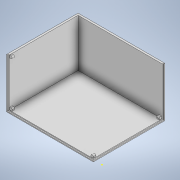
# Autodesk Inventor part: kevnat part1
Saved by Autodesk Inventor 2022 (Build 260153000, 153)
## iProperties
Created: 2023-03-07
Part Number: kevnat part1
Material: Generic
Document SubType Name: Modeling
Designer: Riordan
Density: 1 g/cm^3
Appearance: Default
Author: Riordan
Autodesk Inventor part; units mm, degrees
ref_plane "YZ Plane" through (0, 0, 0) normal (1, 0, 0) x (0, 1, 0)
ref_plane "XZ Plane" through (0, 0, 0) normal (0, 1, 0) x (-1, 0, 0)
sketch "Sketch1" plane through (0, 0, 0) normal (0, 1, 0) x (-1, 0, 0)
  line L0 (0, 0) -> (200, 0)
  line L1 (200, 0) -> (200, -150)
  line L2 (200, -150) -> (0, -150)
  line L3 (0, -150) -> (0, 0)
  dimension "d0" = 200
  dimension "d1" = 150
  constraints: 8 end point, 2 parallel, 1 horizontal, 1 perpendicular
  measures "d0" distance of L1.end L2.end
  measures "d1" distance of L0.end L1.end
extrude "Extrusion1" add sketch "Sketch1" along normal blind 2
sketch "Sketch2" plane through (0, 2, 0) normal (0, 1, 0) x (1, 0, 0)
  line L0 (-200, 0) -> (0, 0) projected
  line L1 (-200, 0) -> (-200, 2)
  line L2 (-200, 150) -> (-200, 0) projected
  line L3 (-200, 2) -> (-2, 2)
  line L4 (-2, 2) -> (-2, 150)
  line L5 (0, 150) -> (-200, 150) projected
  line L6 (-200, 2) -> (-200, 150)
  line L7 (-200, 150) -> (-2, 150)
  dimension "d4" = 2
  dimension "d5" = 198
  constraints: 10 end point, 3 perpendicular, 3 point on line
  measures "d4" distance of L0.start L1.end
  measures "d5" distance of L1.end L3.end
extrude "Extrusion2" add sketch "Sketch2" along normal blind 2
sketch "Sketch3" plane through (0, 4, 0) normal (0, 1, 0) x (1, 0, 0)
  line L0 (0, 0) -> (0, 150) projected
  line L1 (0, 0) -> (-198, 0)
  line L2 (-198, 0) -> (-198, 148)
  line L3 (-198, 148) -> (0, 148)
  line L4 (0, 148) -> (0, 0)
  line L5 (0, 150) -> (-200, 150) projected
  line L6 (-200, 150) -> (0, 150)
  line L7 (0, 150) -> (0, 0)
  line L8 (0, 0) -> (-200, 0)
  line L9 (-200, 0) -> (-200, 150)
  dimension "d8" = 198
  dimension "d9" = 148
  constraints: 16 end point, 4 parallel, 2 horizontal, 2 perpendicular
  measures "d8" distance of L2.end L3.end
  measures "d9" distance of L1.end L2.end
extrude "Extrusion3" add sketch "Sketch3" along normal blind 100 and the other way blind 2 contours L3 L2 L8 L9 L5 L0
sketch "Sketch4" plane through (0, 4, 0) normal (0, 1, 0) x (1, 0, 0)
  line L0 (-198, 2) -> (-2, 2) projected
  line L1 (-198, 2) -> (-196, 2)
  line L2 (-196, 2) -> (-196, 146)
  line L3 (-2, 148) -> (-198, 148) projected
  line L4 (-196, 146) -> (-2, 146)
  line L5 (-2, 2) -> (-2, 148) projected
  line L6 (-2, 2) -> (-198, 2)
  line L7 (-198, 2) -> (-198, 148)
  line L8 (-198, 148) -> (-2, 148)
  line L9 (-2, 148) -> (-2, 2)
  point P0 (0, 0)
  dimension "d14" = 2
  dimension "d15" = 144
  constraints: 14 end point, 3 perpendicular, 2 parallel, 2 point on line, 1 horizontal
  measures "d14" distance of L0.start L1.end
  measures "d15" distance of L1.end L2.end
extrude "Extrusion4" add sketch "Sketch4" along normal blind 100 contours L7 L3 L5 L4 L2 L0
sketch "Sketch7" plane through (0, 4, 0) normal (0, 1, 0) x (1, 0, 0)
  line L0 (-196, 2) -> (-2, 2) projected
  line L1 (-196, 2) -> (-196, 3)
  line L2 (-196, 146) -> (-196, 2) projected
  line L3 (-196, 3) -> (-191, 3)
  line L4 (-191, 3) -> (-191, 8)
  line L5 (-191, 8) -> (-196, 8)
  point P0 (0, 0)
  point P1 (-196, 117.9293)
  dimension "d36" = 1
  dimension "d37" = 5
  dimension "d38" = 5
  constraints: 8 end point, 3 perpendicular, 2 point on line
  measures "d36" distance of L0.start L1.end
  measures "d37" distance of L1.end L3.end
  measures "d38" distance of L3.end L4.end
extrude "Extrusion7" add sketch "Sketch7" along normal blind 5
fillet "Fillet2" radius 2.5 1 edges at (-191, 9, -5.5)
sketch "Sketch9" plane through (0, 4, 0) normal (0, 1, 0) x (1, 0, 0)
  line L0 (-196, 2) -> (-2, 2) projected
  line L1 (-2, 2) -> (-2, 3)
  line L2 (-2, 2) -> (-2, 146) projected
  line L3 (-2, 3) -> (-3, 3)
  line L4 (-3, 3) -> (-8, 3)
  line L5 (-8, 3) -> (-8, 8)
  line L6 (-8, 8) -> (-3, 8)
  line L7 (-3, 8) -> (-3, 3)
  point P0 (0, 0)
  dimension "d45" = 1
  dimension "d46" = 1
  dimension "d47" = 5
  dimension "d48" = 5
  constraints: 12 end point, 2 horizontal, 2 parallel, 1 perpendicular, 1 point on line
  measures "d45" distance of L0.end L1.end
  measures "d46" distance of L1.end L3.end
  measures "d47" distance of L5.end L6.end
  measures "d48" distance of L4.end L5.end
extrude "Extrusion9" add sketch "Sketch9" along normal blind 5
fillet "Fillet3" radius 2.5 2 edges at (-8, 9, -5.5) (-3, 9, -5.5)
sketch "Sketch10" plane through (-8, 4, -3) normal (0, 0, 1) x (1, 0, 0)
  arc A0 (5, 2.5) -> (0, 2.5) centre (2.5, 2.5) ccw projected
  circle A1 centre (2.5, 2.5) radius 1
  point P0 (8, -4)
  dimension "d52" = 2
  constraints: 1 centre point, 1 coincident
  measures "d52" diameter of A1
extrude "Extrusion10" cut sketch "Sketch10" against normal blind 5
sketch "Sketch11" plane through (0, 4, 0) normal (0, 1, 0) x (1, 0, 0)
  line L0 (-2, 146) -> (-196, 146) projected
  line L1 (-2, 146) -> (-3, 146)
  line L2 (-3, 146) -> (-8, 146)
  line L3 (-8, 146) -> (-8, 141)
  line L4 (-8, 141) -> (-3, 141)
  line L5 (-3, 141) -> (-3, 146)
  point P0 (0, 0)
  point P1 (-144.9293, 146)
  dimension "d55" = 1
  dimension "d56" = 5
  dimension "d57" = 5
  constraints: 10 end point, 2 parallel, 1 horizontal, 1 perpendicular, 1 point on line
  measures "d55" distance of L0.start L1.end
  measures "d56" distance of L4.end L3.end
  measures "d57" distance of L3.end L2.end
extrude "Extrusion11" add sketch "Sketch11" along normal blind 5
fillet "Fillet4" radius 2.5 1 edges at (-5.5, 9, -141)
sketch "Sketch12" plane through (-3, 4, -141) normal (1, 0, 0) x (0, 0, -1)
  arc A0 (2.5, 5) -> (0, 2.5) centre (2.5, 2.5) ccw projected
  circle A1 centre (2.5, 2.5) radius 1
  point P0 (-141, -4)
  dimension "d61" = 2
  constraints: 1 centre point, 1 coincident
  measures "d61" diameter of A1
extrude "Extrusion12" cut sketch "Sketch12" against normal blind 5
sketch "Sketch13" plane through (-196, 104, -146) normal (0, 0, 1) x (1, 0, 0)
  line L0 (0, 0) -> (194, 0) projected
  line L1 (194, 0) -> (193, 0)
  line L2 (193, 0) -> (193, -1)
  line L3 (193, -1) -> (188, -1)
  line L4 (188, -1) -> (188, -6)
  line L5 (188, -6) -> (193, -6)
  line L6 (193, -6) -> (193, -1)
  point P0 (196, -104)
  dimension "d64" = 1
  dimension "d65" = 1
  dimension "d66" = 5
  dimension "d67" = 5
  constraints: 12 end point, 2 parallel, 2 perpendicular, 1 horizontal, 1 point on line
  measures "d64" distance of L0.end L1.end
  measures "d65" distance of L1.end L2.end
  measures "d66" distance of L5.end L4.end
  measures "d67" distance of L4.end L3.end
extrude "Extrusion13" add sketch "Sketch13" along normal blind 5
fillet "Fillet5" radius 2.5 2 edges at (-5.5, 103, -141) (-5.5, 98, -141)
sketch "Sketch14" plane through (-3, 98, -146) normal (1, 0, 0) x (0, 0, -1)
  arc A0 (-2.5, 5) -> (-2.5, 0) centre (-2.5, 2.5) ccw projected
  circle A1 centre (-2.5, 2.5) radius 1
  point P0 (-146, -98)
  dimension "d71" = 2
  constraints: 1 centre point, 1 coincident
  measures "d71" diameter of A1
extrude "Extrusion14" cut sketch "Sketch14" against normal blind 5
sketch "Sketch15" plane through (-196, 4, -2) normal (1, 0, 0) x (0, 0, -1)
  line L0 (0, 100) -> (0, -2) projected
  line L1 (0, 100) -> (1, 100)
  line L2 (148, 100) -> (-2, 100) projected
  line L3 (1, 100) -> (1, 99)
  line L4 (1, 99) -> (6, 99)
  line L5 (6, 99) -> (6, 94)
  line L6 (6, 94) -> (1, 94)
  line L7 (1, 94) -> (1, 99)
  point P0 (-2, -4)
  dimension "d74" = 1
  dimension "d75" = 1
  dimension "d76" = 5
  dimension "d77" = 5
  constraints: 12 end point, 2 parallel, 2 perpendicular, 1 horizontal, 1 point on line
  measures "d74" distance of L0.start L1.end
  measures "d75" distance of L1.end L3.end
  measures "d76" distance of L5.end L6.end
  measures "d77" distance of L4.end L5.end
extrude "Extrusion15" add sketch "Sketch15" along normal blind 5
fillet "Fillet6" radius 2.5 2 edges at (-191, 103, -5.5) (-191, 98, -5.5)
sketch "Sketch17" plane through (0, 4, 0) normal (0, 1, 0) x (1, 0, 0)
  point P0 (0, 0)
sketch "Sketch18" plane through (0, 4, 0) normal (0, 1, 0) x (1, 0, 0)
  line L0 (-196, 2) -> (-196, 146) projected
  line L1 (-196, 84.7457) -> (-26, 84.7457)
  line L2 (0, 0) -> (0, 150) projected
  line L3 (-26, 84.7457) -> (-26, 146)
  line L4 (-196, 146) -> (-2, 146) projected
  line L5 (-26, 84.7457) -> (-26, 2)
  line L6 (-196, 2) -> (-2, 2) projected
  line L7 (-26, 143.5) -> (-27, 143.5)
  line L8 (-27, 143.5) -> (-2, 143.5)
  line L9 (-2, 148) -> (-2, 2) projected
  line L10 (-14.5, 143.5) -> (-14.5, 2)
  line L11 (-14.5, 143.5) -> (-16.2266, 143.5)
  line L12 (-16.2266, 143.5) -> (-16.2266, 2)
  line L13 (-16.2266, 2) -> (-14.5, 2)
  line L14 (-14.5, 2) -> (-14.5, 143.5)
  line L15 (-16.2266, 143.5) -> (-14.5, 143.5)
  line L16 (-14.5, 143.5) -> (-14.5, 2)
  line L17 (-14.5, 2) -> (-16.2266, 2)
  line L18 (-16.2266, 2) -> (-16.2266, 143.5)
  dimension "d84" = 170
  dimension "d85" = 1
  constraints: 28 end point, 8 point on line, 5 perpendicular, 4 parallel, 3 horizontal, 1 midpoint, 1 vertical
  measures "d84" distance of L1.start L1.end
  measures "d85" distance of L7.start L7.end
sketch "Sketch19" plane through (0, 4, 0) normal (0, 1, 0) x (1, 0, 0)
  point P0 (0, 0)
extrude "Extrusion17" add sketch "Sketch18" along normal blind 10 contours L12 L8 L10 L6
ref_plane "Work Plane1" through (-14.5, 14, -2) normal (-1, 0, 0) x (0, 0, -1)
mirror "Mirror1" about plane through (-14.5, 4, -2) normal (1, 0, 0) of "Fillet3", "Extrusion9", "Extrusion11", "Fillet4"
sketch "Sketch20" plane through (0, 2, 0) normal (0, 1, 0) x (1, 0, 0)
  line L0 (-26, 143.5) -> (-21, 143.5) projected
  line L1 (-21, 143.5) -> (-20, 143.5)
  line L2 (-8, 146) -> (-21, 146) projected
  line L3 (-2, 148) -> (-2, 2) projected
  line L4 (-20, 146) -> (-2, 146)
  line L5 (-2, 146) -> (-2, 2)
  line L6 (-2, 2) -> (-20, 2)
  line L7 (-20, 2) -> (-20, 146)
  line L8 (0, 148) -> (-2, 148) projected
  line L9 (-20, 2) -> (-2, 2)
  line L10 (-2, 2) -> (-2, 148)
  line L11 (-2, 148) -> (-20, 148)
  line L12 (-20, 148) -> (-20, 2)
  point P0 (0, 0)
  dimension "d88" = 1
  constraints: 18 end point, 4 parallel, 2 horizontal, 2 perpendicular, 1 collinear, 1 point on line
  measures "d88" distance of L0.end L1.end
extrude "Extrusion18" cut sketch "Sketch20" along normal blind 1000
sketch "Sketch21" plane through (0, 2, 0) normal (0, 1, 0) x (1, 0, 0)
  line L0 (-20, 148) -> (-20, 2) projected
  line L1 (-20, 2) -> (-18, 2)
  line L2 (-198, 0) -> (0, 0) projected
  line L3 (0, 150) -> (-200, 150) projected
  line L4 (-18, 0) -> (0, 0)
  line L5 (0, 0) -> (0, 150)
  line L6 (0, 150) -> (-18, 150)
  line L7 (-18, 150) -> (-18, 0)
  dimension "d91" = 2
  constraints: 10 end point, 2 horizontal, 2 parallel, 1 perpendicular, 1 point on line
  measures "d91" distance of L0.end L1.end
extrude "Extrusion19" cut sketch "Sketch21" along normal mid plane 1000
sketch "Sketch23" plane through (0, 4, 0) normal (0, 1, 0) x (1, 0, 0)
  point P0 (0, 0)
body "Solid1"
